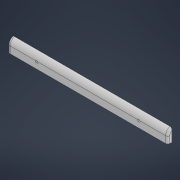
# Autodesk Inventor part: Topo_Aerofoil
Saved by Autodesk Inventor 2022 (Build 260153000, 153)
## iProperties
Created: 2022-06-10
Part Number: Topo_Aerofoil
Material: Generic
Document SubType Name: Modeling
Designer: Gugarauj07
Density: 1 g/cm^3
Appearance: Default
Author: Gugarauj07
Autodesk Inventor part; units mm, degrees
ref_plane "YZ Plane" through (0, 0, 0) normal (1, 0, 0) x (0, 1, 0)
ref_plane "XZ Plane" through (0, 0, 0) normal (0, 1, 0) x (-1, 0, 0)
ref_plane "XY Plane" through (0, 0, 0) normal (0, 0, 1) x (1, 0, 0)
sketch "Sketch1" plane through (0, 0, 0) normal (0, 0, 1) x (1, 0, 0)
  line L0 (-375, 30) -> (375, 30)
  line L1 (375, 30) -> (375, -30)
  line L2 (375, -30) -> (-375, -30)
  line L3 (-375, -30) -> (-375, 30)
  circle A0 centre (-240, 0) radius 5
  circle A1 centre (240, 0) radius 5
  point P0 (0, 0)
  dimension "d0" = 750
  dimension "d1" = 60
  dimension "d3" = 10
  constraints: 8 end point, 2 centre point, 2 parallel, 1 horizontal, 1 perpendicular
  measures "d0" distance of L1.end L2.end
  measures "d1" distance of L0.end L1.end
  measures "d3" diameter of A0
extrude "Extrusion1" add sketch "Sketch1" along normal blind 20
fillet "Fillet1" radius 30 1 edges at (0, 30, 20)
fillet "Fillet2" radius 10 4 edges at (-375, -14.1421, 20) (-375, 19.0362, 14.4949) (375, 19.0362, 14.4949) (375, -14.1421, 20)
body "Solid1"
